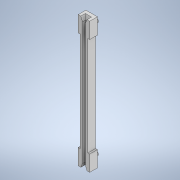
# Autodesk Inventor part: CCA Rail
Saved by Autodesk Inventor 2021 (Build 250183000, 183)
## iProperties
Created: 2022-07-24
Part Number: CCA Rail
Material: Generic
Document SubType Name: Modeling
Designer: erics
Density: 1 g/cm^3
Appearance: Default
Author: erics
Autodesk Inventor part; units mm, degrees
ref_plane "YZ Plane" through (0, 0, 0) normal (1, 0, 0) x (0, 1, 0)
ref_plane "XZ Plane" through (0, 0, 0) normal (0, 1, 0) x (-1, 0, 0)
ref_plane "XY Plane" through (0, 0, 0) normal (0, 0, 1) x (1, 0, 0)
sketch "Sketch1" plane through (0, 0, 0) normal (0, 0, 1) x (1, 0, 0)
  line L0 (0, 0) -> (9.8, 0)
  line L1 (9.8, 0) -> (9.8, 13.6)
  line L2 (9.8, 13.6) -> (0, 13.6)
  line L3 (0, 13.6) -> (0, 0)
  line L4 (1.575, 13.6) -> (8.225, 13.6)
  line L5 (8.225, 13.6) -> (8.225, 98.4)
  line L6 (8.225, 98.4) -> (1.575, 98.4)
  line L7 (1.575, 98.4) -> (1.575, 13.6)
  line L8 (1.575, 56) -> (8.225, 56) construction
  line L9 (0, 112) -> (9.8, 112)
  line L10 (9.8, 112) -> (9.8, 98.4)
  line L11 (9.8, 98.4) -> (0, 98.4)
  line L12 (0, 98.4) -> (0, 112)
  line L13 (1.575, 98.4) -> (8.225, 98.4)
  circle A0 centre (4.9, 6.75) radius 2
  line L14 (4.9, 6.75) -> (4.9, 56) construction
  circle A1 centre (4.9, 105.25) radius 2
  line L15 (4.9, 105.25) -> (4.9, 56) construction
  point P0 (4.9, 13.6)
  point P1 (4.9, 98.4)
  dimension "d0" = 9.8
  dimension "d1" = 13.6
  dimension "d2" = 112
  dimension "d3" = 6.65
  dimension "d6" = 4
  dimension "d7" = 98.5
  constraints: 32 end point, 5 midpoint, 5 symmetric about line, 4 parallel, 2 centre point, 2 horizontal, 2 perpendicular, 2 vertical, 1 collinear, 1 equal radius
  measures "d0" distance of L2.end L1.end
  measures "d1" distance of L1.end L0.end
  measures "d2" distance between parallel lines of L0 L9
  measures "d3" distance between parallel lines of L5 L7
  measures "d6" diameter of A0
  measures "d7" distance of L15.start L14.start
extrude "Extrusion1" add sketch "Sketch1" along normal blind 6.6 contours L3 L2 L1 L0 | L7 L6 L5 L2 | L11 L12 L9 L10 L6 | A0 | A1
extrude "Extrusion2" add sketch "Sketch1" against normal blind 3.75 contours A0 | A1
sketch "Sketch2" plane through (0, 0, 6.6) normal (0, 0, 1) x (1, 0, 0)
  line L0 (0, 0) -> (9.8, 0) projected
  line L1 (3.7, 0) -> (6.1, 0)
  line L2 (6.1, 0) -> (6.1, 112)
  line L3 (6.1, 112) -> (3.7, 112)
  line L4 (3.7, 112) -> (3.7, 0)
  line L5 (9.8, 112) -> (0, 112) projected
  point P0 (4.9, 112)
  dimension "d10" = 2.4
  constraints: 8 end point, 2 midpoint, 2 parallel, 1 horizontal, 1 perpendicular, 1 point on line
  measures "d10" distance between parallel lines of L2 L4
extrude "Extrusion3" cut sketch "Sketch2" against normal blind 2.4
chamfer "Chamfer1" distance 3.5 angle 22.5 1 edges at (3.7, 112, 5.4) measured on face at (3.7, 74.6667, 5.8)
chamfer "Chamfer2" distance 3.5 angle 22.5 1 edges at (6.1, 112, 5.4) measured on face at (6.1, 37.3333, 5.8)
chamfer "Chamfer3" distance 3.5 angle 22.5 1 edges at (4.9, 112, 4.2) measured on face at (4.5, 36.1667, 4.2)
chamfer "Chamfer4" distance 3.5 angle 22.5 1 edges at (3.7, 0, 5.4) measured on face at (3.7, 36.1667, 5)
chamfer "Chamfer5" distance 3.5 angle 22.5 1 edges at (6.1, 0, 5.4) measured on face at (6.1, 36.1667, 5.8)
chamfer "Chamfer6" distance 3.5 angle 22.5 1 edges at (4.9, 0, 4.2) measured on face at (5.3, 73.5, 4.2)
body "Solid1"
